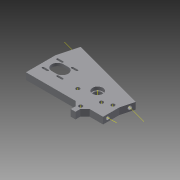
# Autodesk Inventor part: Vertex Bottom tensioner right
Saved by Autodesk Inventor 2013 (Build 170138000, 138)
## iProperties
Created: 2013-01-09
Part Number: Vertex Bottom tensioner right
Material: Generic
Document SubType Name: Modeling
Designer: Nico
Density: 1 g/cm^3
Author: Nico
Autodesk Inventor part; units mm, degrees
ref_plane "YZ Plane" through (0, 0, 0) normal (1, 0, 0) x (0, 1, 0)
ref_plane "XZ Plane" through (0, 0, 0) normal (0, 1, 0) x (-1, 0, 0)
ref_plane "XY Plane" through (0, 0, 0) normal (0, 0, 1) x (1, 0, 0)
sketch "Sketch1" plane through (0, 0, 0) normal (0, 0, 1) x (1, 0, 0)
  line L0 (11.0906, 0.1113) -> (11.0906, 10.1113)
  line L1 (11.0906, 10.1113) -> (1.0906, 20.1113)
  line L2 (31.0918, 20.1126) -> (21.0906, 10.1113)
  line L3 (21.0906, 10.1113) -> (21.0906, 0.1113)
  line L4 (21.0906, 0.1113) -> (11.0906, 0.1113)
  circle A0 centre (16.0906, 16.0413) radius 3.9
  line L5 (37.1863, 89.9817) -> (4.7287, 98.6787)
  line L6 (41.216, 88.9019) -> (37.1863, 89.9817)
  circle A1 centre (31.0906, 45.1113) radius 4
  circle A2 centre (-18.9094, 45.1113) radius 4
  line L7 (1.0906, 20.1113) -> (-38.9094, 20.1113)
  line L8 (4.7287, 98.6787) -> (-28.7852, 107.6587)
  circle A3 centre (6.0906, 62.1113) radius 9
  line L9 (-38.9094, 69.8746) -> (-28.7852, 107.6587)
  line L10 (31.0918, 20.1126) -> (59.4992, 20.1126)
  line L11 (59.4992, 20.1126) -> (59.4992, 54.8735)
  line L12 (59.4992, 84.003) -> (41.216, 88.9019)
  line L13 (59.4992, 54.8735) -> (66.7815, 82.0517)
  line L14 (66.7815, 82.0517) -> (59.4992, 84.003)
  circle A4 centre (48.4066, 52.1126) radius 3.9
  line L15 (-38.9094, 69.8746) -> (-38.9094, 20.1113)
  point P0 (0, 0)
  dimension "d2" = 10
  dimension "d5" = 135
  dimension "d6" = 135
  dimension "d7" = 10
  dimension "d8" = 10
  dimension "d11" = 7.8
  dimension "d14" = 8
  dimension "d15" = 8
  dimension "d16" = 50
  dimension "d20" = 18
  dimension "d21" = 17
  dimension "d24" = 25
  dimension "d30" = 90
  dimension "d31" = 39.117
  dimension "d51" = 7.8
  dimension "d52" = 10
  dimension "d53" = 32
  dimension "d71" = 34.7609
  dimension "d72" = 25
  dimension "d73" = 25
  dimension "d74" = 5
  dimension "d75" = 49.7632
  dimension "d141" = 20
  constraints: 32 end point, 5 centre point, 5 perpendicular, 3 horizontal, 2 parallel, 2 vertical, 1 collinear
  measures "d2" distance between parallel lines of L3 L0
  measures "d5" angle of L0 L1
  measures "d6" angle of L3 L2
  measures "d7" distance of L0.start L0.end
  measures "d8" distance of L2.end L3.end
  measures "d11" diameter of A0
  measures "d14" diameter of A1
  measures "d15" diameter of A2
  measures "d16" distance of A1.centre A2.centre
  measures "d20" diameter of A3
  measures "d21" vertical distance of A3.centre A2.centre
  measures "d24" horizontal distance of A2.centre A3.centre
  measures "d30" angle of L9 L8
  measures "d31" distance of L9.start L8.end
  measures "d51" diameter of A4
  measures "d52" distance from line of A4.centre L13
  measures "d53" distance from line of L10 A4.centre
  measures "d71" distance of L10.end L11.end
  measures "d72" distance from line of L7 A2.centre
  measures "d73" distance from line of L7 A1.centre
  measures "d74" distance from line of L0 A0.centre
  measures "d75" distance of L7.end L9.start
  measures "d141" distance from line of L15 A2.centre
extrude "Extrusion6" add sketch "Sketch1" along normal blind 14
sketch "Sketch6" plane through (59.4992, 20.1126, 0) normal (1, 0, 0) x (0, 0, -1)
  circle A0 centre (-7, 10.2998) radius 3.8217
  line L0 (0, -20.0012) -> (-14, -20.0012) projected
  point P0 (0, -20.1126)
  dimension "d76" = 30.301
  constraints: 1 centre point
  measures "d76" distance from line of L0 A0.centre
sketch "Sketch7" plane through (66.7815, 82.0517, 14) normal (0.9659258, -0.258819, 0) x (0, 0, -1)
  line L0 (14, 0) -> (0, 0) projected
  circle A0 centre (7, -10) radius 3.9
  point P0 (14, -96.5401)
  dimension "d58" = 7.8
  dimension "d60" = 10
  constraints: 1 centre point
  measures "d58" diameter of A0
  measures "d60" distance from line of A0.centre L0
sketch "Sketch9" plane through (0, 0, 14) normal (0, 0, 1) x (1, 0, 0)
  circle A0 centre (-18.9094, 45.1113) radius 4 projected
  circle A1 centre (31.0906, 45.1113) radius 4 projected
  point P0 (0, 0)
extrude "Extrusion10" add sketch "Sketch9" against normal blind 5
sketch "Sketch10" plane through (0, 0, 14) normal (0, 0, 1) x (1, 0, 0)
  circle A0 centre (6.0906, 62.1113) radius 9 projected
  circle A1 centre (6.0906, 62.1113) radius 11
  point P0 (0, 0)
  dimension "d77" = 22
  constraints: 1 centre point, 1 coincident
  measures "d77" diameter of A1
extrude "Extrusion11" cut sketch "Sketch10" against normal blind 7
sketch "Sketch11" plane through (0, 0, 14) normal (0, 0, 1) x (1, 0, 0)
  line L0 (-28.7852, 107.6587) -> (-38.9094, 69.8746) projected
  line L1 (-38.9094, 69.8746) -> (-38.9094, 20.1113) projected
  line L2 (-38.9094, 20.1113) -> (1.0906, 20.1113) projected
  line L3 (-38.9094, 20.1113) -> (-103.9094, 20.1113)
  line L4 (-103.9094, 20.1113) -> (-103.9094, 82.0517)
  line L5 (-28.7852, 107.6587) -> (-92.4753, 124.7244)
  line L6 (-103.9094, 82.0517) -> (-92.4753, 124.7244)
  point P0 (0, 0)
  dimension "d81" = 15
  dimension "d82" = 65
  dimension "d140" = 15
  constraints: 8 end point, 2 perpendicular, 1 collinear
  measures "d81" angle of L3 L5
  measures "d82" distance of L1.end L3.end
  measures "d140" angle of L4 L6
extrude "Extrusion12" add sketch "Sketch11" against normal blind 14
extrude "Extrusion13" cut sketch "Sketch6" against normal blind 300
extrude "Extrusion14" cut sketch "Sketch7" against normal blind 300
sketch "Sketch12" plane through (0, 0, 14) normal (0, 0, 1) x (1, 0, 0)
  circle A0 centre (6.0906, 62.1113) radius 11 projected
  line L0 (1.0906, 20.1113) -> (-103.9094, 20.1113) projected
  arc A1 (-94.4094, 79.6113) -> (-94.4094, 75.6113) centre (-94.4094, 77.6113) ccw
  arc A2 (-94.4094, 48.6113) -> (-94.4094, 44.6113) centre (-94.4094, 46.6113) ccw
  line L1 (-78.9569, 74.554) -> (-68.957, 74.5922)
  line L2 (-78.9569, 49.6686) -> (-68.957, 49.6305)
  arc A3 (-78.9569, 74.554) -> (-78.9569, 49.6686) centre (-78.9094, 62.1113) ccw
  arc A4 (-68.957, 49.6305) -> (-68.957, 74.5922) centre (-68.9094, 62.1113) ccw
  arc A5 (-84.4094, 75.6113) -> (-84.4094, 79.6113) centre (-84.4094, 77.6113) ccw
  arc A6 (-84.4094, 44.6113) -> (-84.4094, 48.6113) centre (-84.4094, 46.6113) ccw
  line L3 (-94.4094, 75.6113) -> (-84.4094, 75.6113)
  line L4 (-84.4094, 79.6113) -> (-94.4094, 79.6113)
  line L5 (-94.4094, 44.6113) -> (-84.4094, 44.6113)
  line L6 (-84.4094, 48.6113) -> (-94.4094, 48.6113)
  arc A7 (-63.4094, 79.6113) -> (-63.4094, 75.6113) centre (-63.4094, 77.6113) ccw
  arc A8 (-53.4094, 75.6113) -> (-53.4094, 79.6113) centre (-53.4094, 77.6113) ccw
  arc A9 (-53.4094, 44.6113) -> (-53.4094, 48.6113) centre (-53.4094, 46.6113) ccw
  arc A10 (-63.4094, 48.6113) -> (-63.4094, 44.6113) centre (-63.4094, 46.6113) ccw
  line L7 (-63.4094, 75.6113) -> (-53.4094, 75.6113)
  line L8 (-53.4094, 79.6113) -> (-63.4094, 79.6113)
  line L9 (-63.4094, 44.6113) -> (-53.4094, 44.6113)
  line L10 (-53.4094, 48.6113) -> (-63.4094, 48.6113)
  point P0 (0, 0)
  dimension "d92" = 42
  dimension "d106" = 42
  dimension "d143" = 85
  dimension "d144" = 75
  dimension "d147" = 10
  dimension "d148" = 10
  dimension "d158" = 4
  dimension "d159" = 4
  dimension "d160" = 4
  dimension "d162" = 15.5
  dimension "d163" = 15.5
  dimension "d166" = 10
  dimension "d167" = 10
  dimension "d168" = 15.5
  dimension "d169" = 15.5
  dimension "d170" = 4
  dimension "d171" = 2
  dimension "d172" = 2
  constraints: 20 end point, 20 point on circle, 10 centre point, 4 horizontal, 4 parallel, 4 tangent
  measures "d92" distance from line of L0 A0.centre
  measures "d106" distance from line of L0 A4.centre
  measures "d143" distance of A0.centre A3.centre
  measures "d144" distance of A0.centre A4.centre
  measures "d147" distance of A2.centre A6.centre
  measures "d148" distance of A1.centre A5.centre
  measures "d158" diameter of A7
  measures "d159" diameter of A10
  measures "d160" diameter of A9
  measures "d162" horizontal distance of A3.centre A7.centre
  measures "d163" horizontal distance of A3.centre A10.centre
  measures "d166" distance of A7.centre A8.centre
  measures "d167" distance of A9.centre A10.centre
  measures "d168" vertical distance of A4.centre A7.centre
  measures "d169" vertical distance of A4.centre A10.centre
  measures "d170" distance between parallel lines of L7 L8
  measures "d171" distance from line of L8 A7.centre
  measures "d172" radius of A8
extrude "Extrusion18" cut sketch "Sketch12" against normal blind 18 contours L4 A5 L3 A1 | L6 A6 L5 A2 | L1 A4 L2 A3 | L8 A8 L7 A7 | L9 A10 L10 A9
sketch "Sketch14" plane through (0, 0, 0) normal (0, 0, -1) x (-1, 0, 0)
  line L0 (63.4094, 44.6113) -> (53.4094, 44.6113) projected
  arc A0 (53.4094, 48.6113) -> (53.4094, 44.6113) centre (53.4094, 46.6113) ccw projected
  line L1 (53.4094, 48.6113) -> (63.4094, 48.6113) projected
  arc A1 (63.4094, 44.6113) -> (63.4094, 48.6113) centre (63.4094, 46.6113) ccw projected
  line L2 (94.4094, 44.6113) -> (84.4094, 44.6113) projected
  arc A2 (84.4094, 48.6113) -> (84.4094, 44.6113) centre (84.4094, 46.6113) ccw projected
  line L3 (84.4094, 48.6113) -> (94.4094, 48.6113) projected
  arc A3 (94.4094, 44.6113) -> (94.4094, 48.6113) centre (94.4094, 46.6113) ccw projected
  line L4 (94.4094, 75.6113) -> (84.4094, 75.6113) projected
  arc A4 (84.4094, 79.6113) -> (84.4094, 75.6113) centre (84.4094, 77.6113) ccw projected
  line L5 (84.4094, 79.6113) -> (94.4094, 79.6113) projected
  arc A5 (94.4094, 75.6113) -> (94.4094, 79.6113) centre (94.4094, 77.6113) ccw projected
  line L6 (63.4094, 75.6113) -> (53.4094, 75.6113) projected
  arc A6 (53.4094, 79.6113) -> (53.4094, 75.6113) centre (53.4094, 77.6113) ccw projected
  line L7 (53.4094, 79.6113) -> (63.4094, 79.6113) projected
  arc A7 (63.4094, 75.6113) -> (63.4094, 79.6113) centre (63.4094, 77.6113) ccw projected
  arc A8 (78.9569, 49.6686) -> (78.9569, 74.554) centre (78.9094, 62.1113) ccw projected
  line L8 (78.9569, 49.6686) -> (68.957, 49.6305) projected
  arc A9 (68.957, 74.5922) -> (68.957, 49.6305) centre (68.9094, 62.1113) ccw projected
  line L9 (68.957, 74.5922) -> (78.9569, 74.554) projected
  line L10 (51.4094, 39.6113) -> (96.4094, 39.6113)
  line L11 (101.4094, 44.6113) -> (101.4094, 79.6113)
  line L12 (96.4094, 84.6113) -> (51.4094, 84.6113)
  line L13 (46.4094, 79.6113) -> (46.4094, 44.6113)
  arc A10 (101.4094, 79.6113) -> (96.4094, 84.6113) centre (96.4094, 79.6113) ccw
  arc A11 (51.4094, 84.6113) -> (46.4094, 79.6113) centre (51.4094, 79.6113) ccw
  arc A12 (46.4094, 44.6113) -> (51.4094, 39.6113) centre (51.4094, 44.6113) ccw
  arc A13 (96.4094, 39.6113) -> (101.4094, 44.6113) centre (96.4094, 44.6113) ccw
  point P0 (0, 0)
  dimension "d175" = 45
  dimension "d177" = 22.5
  dimension "d178" = 55
  dimension "d179" = 22.5
  dimension "d180" = 5
  constraints: 8 end point, 8 point on circle, 8 tangent, 4 centre point, 3 equal radius, 2 parallel, 1 horizontal, 1 perpendicular
  measures "d175" distance between parallel lines of L12 L10
  measures "d177" distance from line of L10 A9.centre
  measures "d178" distance between parallel lines of L11 L13
  measures "d179" distance from line of L13 A9.centre
  measures "d180" radius of A10
extrude "Extrusion19" cut sketch "Sketch14" against normal blind 8
sketch "Sketch15" plane through (0, 0, 0) normal (0, 0, -1) x (-1, 0, 0)
  circle A0 centre (18.9094, 45.1113) radius 4 projected
  circle A1 centre (-31.0906, 45.1113) radius 4 projected
  point P0 (0, 0)
extrude "Extrusion20" cut sketch "Sketch15" against normal blind 16
sketch "Sketch16" plane through (0, 0, 0) normal (0, 0, -1) x (-1, 0, 0)
  circle A0 centre (18.9094, 45.1113) radius 4 projected
  circle A1 centre (-31.0906, 45.1113) radius 4 projected
  point P0 (0, 0)
extrude "Extrusion21" add sketch "Sketch16" against normal blind 4
body "Solid2"
